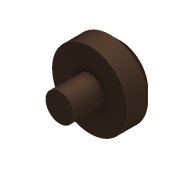
# Autodesk Inventor part: MUSAB5
Saved by Autodesk Inventor 2017 (Build 210142000, 142)
## iProperties
Created: 2017-09-15
Part Number: MUSAB5
Material: Bronze, Soft Tin
Document SubType Name: Modeling
Designer: Amer Mohia
Density: 8.874 g/cm^3
Appearance: Bronze - Satin
Author: Amer Mohia
Autodesk Inventor part; units mm, degrees
ref_plane "YZ Plane" through (0, 0, 0) normal (1, 0, 0) x (0, 1, 0)
ref_plane "XZ Plane" through (0, 0, 0) normal (0, 1, 0) x (-1, 0, 0)
ref_plane "XY Plane" through (0, 0, 0) normal (0, 0, 1) x (1, 0, 0)
sketch "Sketch1" plane through (0, 0, 0) normal (0, 0, 1) x (1, 0, 0)
  line L0 (5.1012, -1.9833) -> (5.1012, -4.9833)
  line L1 (7.4512, -1.9833) -> (7.4512, 0.0167)
  line L2 (4.9512, 1.0167) -> (4.9512, -0.9833)
  line L3 (4.2012, 0.0167) -> (4.2012, -0.9833)
  line L4 (4.9512, 1.0167) -> (6.4512, 1.0167)
  line L5 (7.4512, -1.9833) -> (5.1012, -1.9833)
  line L6 (5.1012, -4.9833) -> (3.7012, -4.9833)
  line L7 (3.7012, -4.9833) -> (3.7012, 0.0167)
  line L8 (4.2012, -0.9833) -> (4.9512, -0.9833)
  line L9 (6.4512, 1.0167) -> (7.4512, 0.0167)
  line L10 (3.7012, 0.0167) -> (4.2012, 0.0167)
  constraints: 22 end point, 4 vertical, 2 horizontal, 1 horizontal alignment, 1 parallel, 1 perpendicular
revolve "Revolution1" add sketch "Sketch1" angle 360 about axis through (3.7012, -4.9833, 0) along (0, 1, 0)
body "Solid1"
